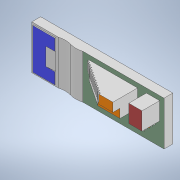
# Autodesk Inventor part: Terrain2021
Saved by Autodesk Inventor 2021 (Build 250183000, 183)
## iProperties
Created: 2021-10-04
Part Number: Terrain2021
Material: 一般
Document SubType Name: Modeling
Designer: tazak
Density: 1 g/cm^3
Appearance: 既定
Author: tazak
Autodesk Inventor part; units mm, degrees
ref_plane "YZ Plane" through (0, 0, 0) normal (1, 0, 0) x (0, 1, 0)
ref_plane "XZ Plane" through (0, 0, 0) normal (0, 1, 0) x (-1, 0, 0)
ref_plane "XY Plane" through (0, 0, 0) normal (0, 0, 1) x (1, 0, 0)
sketch "スケッチ1" plane through (0, 0, 0) normal (0, 0, 1) x (1, 0, 0)
  line L0 (-1000, 2500) -> (14000, 2500)
  line L1 (14000, 2500) -> (14000, -2500)
  line L2 (14000, -2500) -> (-1000, -2500)
  line L3 (-1000, -2500) -> (-1000, 2500)
  line L4 (0, 3500) -> (0, -3500) projected
  point P0 (0, 0)
  point P1 (-1000, 0)
  dimension "d0" = 5000
  dimension "d1" = 1000
  dimension "d2" = 15000
  constraints: 8 end point, 2 parallel, 1 horizontal, 1 horizontal alignment, 1 midpoint, 1 perpendicular
  measures "d0" distance of L2.end L0.start
  measures "d1" distance between parallel lines of L4 L3
  measures "d2" distance of L0.start L0.end
extrude "押し出し1" add sketch "スケッチ1" against normal blind 1000
sketch "スケッチ2" plane through (0, 0, 0) normal (0, 0, 1) x (1, 0, 0)
  line L0 (12000, 2000) -> (13500, 2000)
  line L1 (13500, 2000) -> (13500, 0)
  line L2 (13500, 0) -> (12000, 0)
  line L3 (12000, 0) -> (12000, 2000)
  line L4 (14000, 2500) -> (-1000, 2500) projected
  line L5 (14000, -2500) -> (14000, 2500) projected
  point P0 (0, 0)
  dimension "d31" = 1500
  dimension "d32" = 2000
  dimension "d72" = 500
  dimension "d73" = 500
  constraints: 8 end point, 2 parallel, 1 horizontal, 1 perpendicular
  measures "d31" distance of L0.start L0.end
  measures "d32" distance of L0.end L1.end
  measures "d72" distance between parallel lines of L4 L0
  measures "d73" distance between parallel lines of L5 L1
extrude "押し出し2" add sketch "スケッチ2" along normal blind 2000
sketch "スケッチ3" plane through (0, 0, 0) normal (0, 0, 1) x (1, 0, 0)
  line L0 (5500, 2000) -> (11000, 2000)
  line L1 (11000, 2000) -> (11000, 0)
  line L2 (11000, 0) -> (5500, 0)
  line L3 (5500, 0) -> (5500, 2000)
  line L4 (12000, 2000) -> (12000, 0) projected
  point P0 (0, 0)
  dimension "d28" = 1000
  dimension "d35" = 2000
  dimension "d71" = 5500
  constraints: 8 end point, 2 parallel, 1 horizontal, 1 horizontal alignment, 1 perpendicular
  measures "d28" distance between parallel lines of L4 L1
  measures "d35" distance of L2.end L0.start
  measures "d71" distance of L0.start L0.end
extrude "押し出し3" add sketch "スケッチ3" along normal blind 2000
sketch "スケッチ4" plane through (5500, 0, 0) normal (0, -1, 0) x (1, 0, 0)
  line L0 (0, 0) -> (3000, 2000)
  line L1 (3000, 2000) -> (0, 2000)
  line L2 (0, 2000) -> (0, 0)
  line L3 (0, 0) -> (0, 2000) projected
  line L4 (-6500, 0) -> (8500, 0) projected
  point P0 (-5500, 0)
  dimension "d23" = 3000
  constraints: 6 end point, 2 point on line, 1 coincident, 1 horizontal
  measures "d23" horizontal distance of L0.start L0.end
extrude "押し出し4" cut sketch "スケッチ4" against normal blind 1000
sketch "スケッチ5" plane through (12000, 0, 0) normal (-1, 0, 0) x (0, 0, 1)
  circle A0 centre (1728.0975, -100) radius 40
  circle A1 centre (1428.0975, -100) radius 40
  circle A2 centre (1128.0975, -100) radius 40
  circle A3 centre (828.0975, -100) radius 40
  circle A4 centre (528.0975, -100) radius 40
  line L0 (0, 0) -> (2000, 0) projected
  line L1 (0, 2500) -> (0, -2500) projected
  point P0 (0, 0)
  dimension "d11" = 80
  dimension "d12" = 80
  dimension "d13" = 80
  dimension "d14" = 80
  dimension "d15" = 80
  dimension "d16" = 300
  dimension "d17" = 300
  dimension "d18" = 300
  dimension "d19" = 300
  dimension "d20" = 100
  dimension "d82" = 528.0975
  constraints: 5 centre point, 4 horizontal alignment
  measures "d11" diameter of A1
  measures "d12" diameter of A2
  measures "d13" diameter of A3
  measures "d14" diameter of A4
  measures "d15" diameter of A0
  measures "d16" distance of A1.centre A0.centre
  measures "d17" distance of A2.centre A1.centre
  measures "d18" distance of A3.centre A2.centre
  measures "d19" distance of A4.centre A3.centre
  measures "d20" distance from line of L0 A0.centre
  measures "d82" distance from line of L1 A4.centre
extrude "押し出し5" add sketch "スケッチ5" against normal blind 1500
sketch "スケッチ6" plane through (5500, 1000, 0) normal (0, -1, 0) x (1, 0, 0)
  line L0 (0, 0) -> (0, 2000) projected
  line L1 (0, 200) -> (300, 200)
  line L2 (300, 200) -> (300, 400)
  line L3 (300, 400) -> (600, 400)
  line L4 (600, 400) -> (600, 600)
  line L5 (600, 600) -> (900, 600)
  line L6 (900, 600) -> (900, 800)
  line L7 (900, 800) -> (1200, 800)
  line L8 (1200, 800) -> (1200, 1000)
  line L9 (1200, 1000) -> (1500, 1000)
  line L10 (1500, 1000) -> (1500, 1200)
  line L11 (1500, 1200) -> (1800, 1200)
  line L12 (1800, 1200) -> (1800, 1400)
  line L13 (1800, 1400) -> (2100, 1400)
  line L14 (2100, 1400) -> (2100, 1600)
  line L15 (2100, 1600) -> (2400, 1600)
  line L16 (2400, 1600) -> (2400, 1800)
  line L17 (2400, 1800) -> (2700, 1800)
  line L18 (2700, 1800) -> (2700, 2000)
  line L19 (2700, 2000) -> (0, 2000)
  line L20 (0, 2000) -> (0, 200)
  line L21 (-6500, 0) -> (8500, 0) projected
  point P0 (-5500, 0)
  dimension "d46" = 200
  dimension "d47" = 300
  dimension "d48" = 200
  dimension "d49" = 300
  dimension "d50" = 200
  dimension "d51" = 300
  dimension "d52" = 200
  dimension "d53" = 300
  dimension "d54" = 200
  dimension "d55" = 300
  dimension "d56" = 200
  dimension "d57" = 300
  dimension "d58" = 200
  dimension "d59" = 300
  dimension "d60" = 200
  dimension "d61" = 300
  dimension "d62" = 200
  dimension "d63" = 300
  constraints: 40 end point, 19 perpendicular, 1 horizontal, 1 point on line
  measures "d46" distance between parallel lines of L21 L1
  measures "d47" distance of L1.start L1.end
  measures "d48" distance of L1.end L2.end
  measures "d49" distance of L2.end L3.end
  measures "d50" distance of L3.end L4.end
  measures "d51" distance of L4.end L5.end
  measures "d52" distance of L5.end L6.end
  measures "d53" distance of L6.end L7.end
  measures "d54" distance of L7.end L8.end
  measures "d55" distance of L8.end L9.end
  measures "d56" distance of L9.end L10.end
  measures "d57" distance of L10.end L11.end
  measures "d58" distance of L11.end L12.end
  measures "d59" distance of L12.end L13.end
  measures "d60" distance of L13.end L14.end
  measures "d61" distance of L14.end L15.end
  measures "d62" distance of L15.end L16.end
  measures "d63" distance of L16.end L17.end
extrude "押し出し6" cut sketch "スケッチ6" against normal blind 1500
sketch "スケッチ7" plane through (0, 0, 0) normal (0, 0, 1) x (1, 0, 0)
  line L0 (-800, 2300) -> (1700, 2300)
  line L1 (1700, 2300) -> (1700, -2300)
  line L2 (1700, -2300) -> (-800, -2300)
  line L3 (-800, -2300) -> (-800, 2300)
  line L4 (-1000, 2500) -> (-1000, -2500) projected
  line L5 (14000, 2500) -> (-1000, 2500) projected
  line L6 (-1000, -2500) -> (14000, -2500) projected
  point P0 (0, 0)
  dimension "d74" = 200
  dimension "d75" = 200
  dimension "d76" = 200
  dimension "d77" = 2500
  constraints: 8 end point, 2 parallel, 1 horizontal, 1 perpendicular
  measures "d74" distance between parallel lines of L3 L4
  measures "d75" distance between parallel lines of L5 L0
  measures "d76" distance between parallel lines of L6 L2
  measures "d77" distance of L0.start L0.end
extrude "押し出し7" add sketch "スケッチ7" along normal blind 100
sketch "スケッチ8" plane through (5500, 1000, 0) normal (0, -1, 0) x (1, 0, 0)
  line L0 (3000, 2000) -> (3000, 2200)
  line L1 (3000, 2200) -> (3300, 2200)
  line L2 (3300, 2200) -> (3300, 2400)
  line L3 (3300, 2400) -> (3600, 2400)
  line L4 (3600, 2400) -> (3600, 2600)
  line L5 (3600, 2600) -> (3900, 2600)
  line L6 (3900, 2600) -> (3900, 2800)
  line L7 (3900, 2800) -> (4177.5018, 2800)
  line L8 (4177.5018, 2800) -> (5500, 2800)
  line L9 (5500, 2000) -> (2700, 2000) projected
  line L10 (5500, 2800) -> (5500, 2000)
  line L11 (5500, 2000) -> (3000, 2000)
  point P0 (-5500, 0)
  point P1 (3020.6908, 2000)
  dimension "d64" = 200
  dimension "d65" = 300
  dimension "d66" = 200
  dimension "d67" = 300
  dimension "d68" = 200
  dimension "d69" = 300
  dimension "d70" = 200
  constraints: 22 end point, 9 perpendicular, 2 point on line, 1 vertical
  measures "d64" distance of L0.start L0.end
  measures "d65" distance of L0.end L1.end
  measures "d66" distance of L1.end L2.end
  measures "d67" distance of L2.end L3.end
  measures "d68" distance of L3.end L4.end
  measures "d69" distance of L4.end L5.end
  measures "d70" distance of L5.end L6.end
extrude "押し出し8" add sketch "スケッチ8" against normal blind 1000
sketch "スケッチ9" plane through (0, 0, 0) normal (0, 1, 0) x (-1, 0, 0)
  line L0 (-1700, 0) -> (-1700, 100) projected
  line L1 (-1700, 0) -> (-700, 100)
  line L2 (-700, 100) -> (-1700, 100)
  line L3 (-1700, 100) -> (-1700, 0)
  point P0 (0, 0)
  dimension "d78" = 1000
  constraints: 6 end point, 1 collinear, 1 perpendicular
  measures "d78" distance of L1.end L0.end
extrude "押し出し9" cut sketch "スケッチ9" along normal mid plane 2000
sketch "スケッチ11" plane through (-1000, -2500, 0) normal (0, -1, 0) x (1, 0, 0)
  circle A0 centre (3700, 2400) radius 2500
  line L0 (0, 0) -> (15000, 0) projected
  line L1 (2700, 0) -> (2700, 100) projected
  line L2 (4400, 0) -> (3000, 0)
  line L3 (3247.7684, -100) -> (4192.4958, -100) construction
  point P0 (1000, 0)
  dimension "d36" = 5000
  dimension "d38" = 2400
  dimension "d79" = 1000
  dimension "d80" = 1400
  dimension "d81" = 100
  constraints: 4 end point, 2 point on circle, 2 point on line, 1 centre point, 1 horizontal, 1 tangent
  measures "d36" diameter of A0
  measures "d38" distance from line of A0.centre L0
  measures "d79" distance from line of A0.centre L1
  measures "d80" distance of L2.start L2.end
  measures "d81" distance between parallel lines of L3 L0
extrude "押し出し10" cut sketch "スケッチ11" against normal through all
sketch "スケッチ12" plane through (-1000, -2500, -1000) normal (0, -1, 0) x (1, 0, 0)
  arc A0 (7171.2315, 0) -> (3028.7685, 0) centre (5100, -1400) ccw
  arc A1 (3000, 1000) -> (4400, 1000) centre (3700, 3400) ccw projected
  line L0 (4400, 1000) -> (15000, 1000) projected
  line L1 (15000, 0) -> (0, 0) projected
  line L2 (7171.2315, 0) -> (3028.7685, 0)
  point P0 (1000, 1000)
  dimension "d42" = 5000
  dimension "d43" = 2400
  constraints: 2 end point, 2 point on circle, 2 point on line, 1 centre point, 1 equal radius
  measures "d42" diameter of A0
  measures "d43" distance from line of A0.centre L0
extrude "押し出し11" add sketch "スケッチ12" against normal blind 5000
